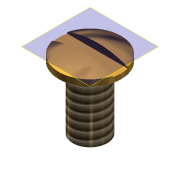
# Autodesk Inventor part: 6-32bolt
Saved by Autodesk Inventor 2022 (Build 260148000, 148)
## iProperties
Shininess: 64.0
Length Units: 11272
Angle Units: 11279
Time Units: 11290
Mass Units: 11286
Length Display Precision: 3
Angle Display Precision: 2
Created: 2002-05-01
Part Number: 6-32bolt
Material: Brass, Soft Yellow
Document SubType Name: Modeling
Designer: Administrator
Density: 8.47 g/cm^3
Appearance: Brass - Satin
Density: 8.47
Volumn: 0.08634729740819558
Area: 1.5307257901253095
PropertySet Name: Model Information
Control State: 0
Master: False
Checked Out: False
Author: Administrator
Autodesk Inventor part; units mm, degrees
ref_plane "YZ Plane" through (0, 0, 0) normal (1, 0, 0) x (0, 1, 0)
ref_plane "XZ Plane" through (0, 0, 0) normal (0, 1, 0) x (-1, 0, 0)
ref_plane "XY Plane" through (0, 0, 0) normal (0, 0, 1) x (1, 0, 0)
sketch "Sketch1" plane through (0, 0, 0) normal (0, 0, 1) x (1, 0, 0)
  line L0 (-17.0246, -1.3061) -> (-17.0246, -8.9261)
  line L1 (-17.0246, -8.9261) -> (-15.272, -8.9261)
  line L2 (-15.272, -8.9261) -> (-15.272, -2.5761)
  line L3 (-15.272, -2.5761) -> (-13.8496, -2.5761)
  line L4 (-13.8496, -2.5761) -> (-13.8496, -1.9411)
  arc A0 (-13.8496, -1.9411) -> (-17.0246, -1.3061) centre (-17.0246, -9.5611) ccw
  dimension "length" = 6.35
  dimension "d1" = 0.635
  dimension "d2" = 1.27
  dimension "d3" = 1.7526
  dimension "d4" = 3.175
  constraints: 10 end point, 3 parallel, 2 point on circle, 1 centre point, 1 perpendicular, 1 vertical, 1 vertical alignment
  measures "length" distance of L1.end L2.end
  measures "d1" distance of L3.end L4.end
  measures "d2" vertical distance of L0.start L2.end
  measures "d3" distance of L0.end L1.end
  measures "d4" horizontal distance of L4.end L0.start
revolve "Revolution1" add sketch "Sketch1" angle 360 about axis through (-17.0246, -1.3061, 0) along (0, -1, 0)
ref_plane "Work Plane1" through (-17.0246, -1.3061, 0) normal (0, -1, 0) x (1, 0, 0)
sketch "Sketch2" plane through (-17.0246, -1.3061, 0) normal (0, -1, 0) x (1, 0, 0)
  line L0 (-3.0822, -0.762) -> (3.0822, -0.762)
  circle A0 centre (0, 0) radius 0.762 construction
  circle A1 centre (0, 0) radius 3.175 projected
  line L1 (-3.0822, 0.762) -> (3.0822, 0.762)
  dimension "d8" = 1.524
  constraints: 4 end point, 4 point on circle, 2 horizontal, 2 tangent, 1 centre point, 1 concentric
  measures "d8" distance from line of L1.start L0
extrude "Extrusion1" cut sketch "Sketch2" along normal blind 0.762 contours A1 L1 L0
thread "Thread1" size "6-32 UNC" class "2A" standard "ANSI Unified Screw Threads" full length
body "Solid1"
